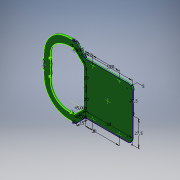
# Autodesk Inventor part: mainpcb
Saved by Autodesk Inventor 2016 (Build 200138000, 138)
## iProperties
Created: 2017-05-27
Part Number: mainpcb
Material: Ogólny
Document SubType Name: Modeling
Designer: Karol
Density: 1 g/cm^3
Appearance: Smooth - Dark Forest Green
Author: Karol
Autodesk Inventor part; units mm, degrees
ref_plane "YZ Plane" through (0, 0, 0) normal (1, 0, 0) x (0, 1, 0)
ref_plane "XZ Plane" through (0, 0, 0) normal (0, 1, 0) x (-1, 0, 0)
ref_plane "XY Plane" through (0, 0, 0) normal (0, 0, 1) x (1, 0, 0)
sketch "Sketch1" plane through (0, 0, 0) normal (0, 1, 0) x (-1, 0, 0)
  line L0 (0, 0) -> (0, -22.5)
  line L1 (0, 0) -> (0, 22.5)
  line L2 (5, 27.5) -> (50, 27.5)
  line L3 (5, -27.5) -> (50, -27.5)
  line L4 (50, 27.5) -> (60.6066, 38.1066)
  line L5 (50, 27.5) -> (65, 27.5) construction
  line L6 (50, -27.5) -> (60.6066, -38.1066)
  line L7 (50, -27.5) -> (65, -27.5) construction
  line L8 (95, 0) -> (95, -5)
  line L9 (95, 0) -> (95, 5)
  arc A0 (5, 27.5) -> (0, 22.5) centre (5, 22.5) ccw
  arc A1 (0, -22.5) -> (5, -27.5) centre (5, -22.5) ccw
  line L10 (60.6066, 38.1066) -> (62.6066, 38.1066)
  line L11 (60.6066, -38.1066) -> (62.6066, -38.1066)
  spline S0 degree 4 poles (62.6066, 38.1066) (69.2667, 38.1066) (82.5868, 38.1066) (95, 24.8465) (95, 11.6155) (95, 5) knots 0 0 0 0 0 0.5 1 1 1 1 1
  spline S1 degree 4 poles (95, -5) (95, -11.6155) (95, -24.8465) (82.5868, -38.1066) (69.2667, -38.1066) (62.6066, -38.1066) knots 0 0 0 0 0 0.5 1 1 1 1 1
  line L12 (52, 0) -> (52, -20)
  line L13 (52, 0) -> (52, 20)
  line L14 (52, 20) -> (62.6066, 30.6066)
  line L15 (52, -20) -> (62.6066, -30.6066)
  line L16 (52, -20) -> (67, -20) construction
  line L17 (62.6066, 30.6066) -> (65.6066, 30.6066)
  line L18 (62.6066, -30.6066) -> (65.6066, -30.6066)
  line L19 (88, 0) -> (88, -8)
  line L20 (88, 0) -> (88, 9)
  spline S2 degree 4 poles (62.6066, 30.6066) (67.2711, 30.6066) (76.6001, 30.6066) (88, 23.7035) (88, 13.9012) (88, 9) knots 0 0 0 0 0 0.5 1 1 1 1 1
  spline S3 degree 4 poles (65.6066, -30.6066) (70.1733, -30.6066) (79.3067, -30.6066) (88, -21.6601) (88, -12.5534) (88, -8) knots 0 0 0 0 0 0.5 1 1 1 1 1
  point P0 (0, -27.5)
  point P1 (0, 27.5)
  point P2 (80, 0)
  point P3 (42, -25)
  point P4 (14, -25)
  point P5 (42, 25)
  point P6 (14, 25)
  point P7 (26, 0)
  dimension "d1" = 27.5
  dimension "d2" = 27.5
  dimension "d3" = 50
  dimension "d4" = 50
  dimension "d5" = 15
  dimension "d6" = 45
  dimension "d7" = 15
  dimension "d8" = 45
  dimension "d17" = 5
  dimension "d18" = 5
  dimension "d19" = 5
  dimension "d20" = 2
  dimension "d21" = 2
  dimension "d22" = 20
  dimension "d23" = 20
  dimension "d24" = 15
  dimension "d25" = 15
  dimension "d26" = 45
  dimension "d27" = 3
  dimension "d28" = 3
  dimension "d29" = 8
  dimension "d30" = 9
  dimension "d40" = 8
  dimension "d41" = 28
  dimension "d42" = 8
  dimension "d43" = 28
  constraints: 42 end point, 13 horizontal, 12 vertical, 4 point on circle, 4 point on line, 4 tangent, 3 equal length, 2 centre point, 1 equal radius, 1 parallel, 8 other
  measures "d1" distance of L0.start point (0, -27.5)
  measures "d2" distance of L0.start point (0, 27.5)
  measures "d3" distance of point (0, 27.5) L2.end
  measures "d4" distance of point (0, -27.5) L3.end
  measures "d5" distance of L2.end L4.end
  measures "d6" angle of L5 L4
  measures "d7" distance of L3.end L6.end
  measures "d8" angle of L6 L7
  measures "d17" distance of L8.start L8.end
  measures "d18" distance of L8.start L9.end
  measures "d19" radius of A0
  measures "d20" distance of L4.end L10.end
  measures "d21" distance of L6.end L11.end
  measures "d22" distance of L12.start L12.end
  measures "d23" distance of L12.start L13.end
  measures "d24" distance of L13.end L14.end
  measures "d25" distance of L12.end L15.end
  measures "d26" angle of L15 L16
  measures "d27" distance of L14.end L17.end
  measures "d28" distance of L15.end L18.end
  measures "d29" distance of L19.start L19.end
  measures "d30" distance of L19.start L20.end
  measures "d40" horizontal distance of point (42, -25) L3.end
  measures "d41" distance of point (42, -25) point (14, -25)
  measures "d42" horizontal distance of L2.end point (42, 25)
  measures "d43" distance of point (14, 25) point (42, 25)
extrude "Extrusion1" add sketch "Sketch1" along normal blind 1.4
hole "Hole1" at (-42, 0, -25) at (-14, 0, -25) at (-42, 0, 25) at (-14, 0, 25) direction (0, 1, 0) diameter 2 depth 2 tip angle 118
body "Solid1"
